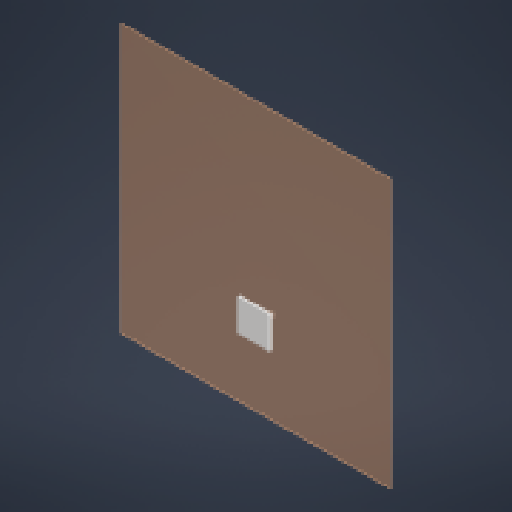
# Autodesk Inventor part: LedMatrix_WS2812_5x5
Saved by Autodesk Inventor 2023.1 (Build 271208000, 208)
## iProperties
Created: 2023-08-25
Part Number: LedMatrix_WS2812_5x5
Material: Generic
Document SubType Name: Modeling
Designer: washichi
Density: 1 g/cm^3
Appearance: Default
Author: washichi
Autodesk Inventor part; units mm, degrees
ref_plane "YZ Plane" through (0, 0, 0) normal (1, 0, 0) x (0, 1, 0)
ref_plane "XZ Plane" through (0, 0, 0) normal (0, 1, 0) x (-1, 0, 0)
ref_plane "XY Plane" through (0, 0, 0) normal (0, 0, 1) x (1, 0, 0)
ref_plane "Work Plane1" through (150.8236, 79.5908, -131.5756) normal (0, 0, 1) x (1, 0, 0)
ref_plane "Work Plane2" through (150.8236, 79.5908, -131.5756) normal (0, 0, 1) x (1, 0, 0)
sketch "Sketch1" plane through (150.8236, 79.5908, -131.5756) normal (0, 0, 1) x (1, 0, 0)
  line L0 (0, 0) -> (0, -70)
  line L1 (-19.45, -89.45) -> (19.45, -89.45)
  line L2 (19.45, -89.45) -> (19.45, -50.55)
  line L3 (19.45, -50.55) -> (-19.45, -50.55)
  line L4 (-19.45, -50.55) -> (-19.45, -89.45)
  line L5 (-19.45, -89.45) -> (19.45, -50.55) construction
  line L6 (19.45, -89.45) -> (-19.45, -50.55) construction
  point P0 (-150.8236, -79.5908)
  dimension "d3" = 70
  dimension "d4" = 38.9
  dimension "d5" = 38.9
  constraints: 14 end point, 2 midpoint, 2 parallel, 1 horizontal, 1 perpendicular, 1 vertical
  measures "d3" distance of L0.start L0.end
  measures "d4" distance of L3.end L2.end
  measures "d5" distance of L2.end L1.end
extrude "Extrusion1" add sketch "Sketch1" along normal blind 3
sketch "Sketch2" plane through (150.8236, 79.5908, -131.5756) normal (0, 0, -1) x (-1, 0, 0)
  line L0 (-17.45, -52.55) -> (-12.45, -52.55)
  line L1 (-12.45, -52.55) -> (-12.45, -57.55)
  line L2 (-12.45, -57.55) -> (-17.45, -57.55)
  line L3 (-17.45, -57.55) -> (-17.45, -52.55)
  line L4 (-17.45, -52.55) -> (-12.45, -57.55) construction
  line L5 (-12.45, -52.55) -> (-17.45, -57.55) construction
  line L6 (-19.45, -89.45) -> (-19.45, -50.55) projected
  line L7 (-19.45, -50.55) -> (19.45, -50.55) projected
  point P0 (150.8236, -79.5908)
  point P1 (-14.95, -55.05)
  dimension "d8" = 5
  dimension "d9" = 5
  dimension "d18" = 2
  dimension "d19" = 2
  constraints: 12 end point, 2 midpoint, 2 parallel, 1 horizontal, 1 perpendicular
  measures "d8" distance of L1.end L2.end
  measures "d9" distance of L0.end L1.end
  measures "d18" distance between parallel lines of L6 L3
  measures "d19" distance between parallel lines of L0 L7
extrude "Extrusion2" add sketch "Sketch2" along normal blind 3
pattern_linear "Rectangular Pattern1" count 5 spacing 7.5 along (-1, 0, 0) count 5 spacing 7.5 along (0, -1, 0) of "Extrusion2"
body "Solid1"
